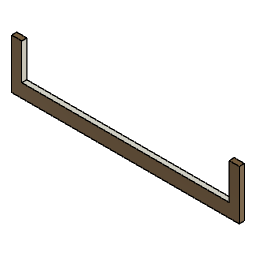
front_panel (Autodesk Fusion 360 design; units mm, degrees)
Autodesk Fusion 360 part; units mm, degrees
note: some values were not read from the file. Set by a fixed rule: which sketch regions a step uses.
sketch "Front Panel" plane through (0, 0, 0) normal (0, 1, 0) x (1, 0, 0)
  line L0 (0, 0) -> (270, 0)
  line L1 (270, 0) -> (270, -30)
  line L2 (258, -16) -> (12, -16)
  line L3 (0, -59) -> (0, 0)
  line L4 (12, -16) -> (12, -59)
  line L5 (12, -59) -> (0, -59)
  line L6 (258, -16) -> (258, -59)
  line L7 (258, -59) -> (270, -59)
  line L8 (270, -59) -> (270, -30)
  dimension "d1" = 270
  dimension "d3" = 43
  dimension "d4" = 12
  dimension "d5" = 12
  dimension "d10" = 16
  dimension "d11" = 43
  constraint horizontal L0
  constraint vertical L1
  constraint horizontal L2
  constraint vertical L3
  constraint coincident L0.start L3.end
  constraint vertical L4
  constraint horizontal L5
  constraint vertical L6
  constraint horizontal L7
  constraint vertical L8
  measures "d1" distance of L0.start L0.end
  measures "d3" distance of L2.end L4.end
  measures "d4" distance of L6.end L7.end
  measures "d5" distance of L4.end L3.start
  measures "d10" distance of L0 L2
  measures "d11" distance of L2 L7
extrude "Extrude1" add sketch "Front Panel" along normal blind 6
equation "mdfThickness = 6 mm" comment "Thickness of the MDF board"
equation "d7 = mdfThickness"
equation "d10 = 10 mm + mdfThickness"
named bodies: "Front Panel"
